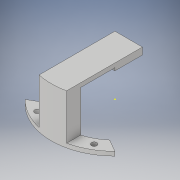
# Autodesk Inventor part: Corona_Cam_Setup_Tool._v2ipt
Saved by Autodesk Inventor 2018 (Build 220112000, 112)
## iProperties
Created: 2020-03-25
Part Number: Corona_Cam_Setup_Tool._v2ipt
Material: Generic
Document SubType Name: Modeling
Designer: Ian
Density: 1 g/cm^3
Appearance: Default
Author: Ian
Autodesk Inventor part; units mm, degrees
ref_plane "YZ Plane" through (0, 0, 0) normal (1, 0, 0) x (0, 1, 0)
ref_plane "XZ Plane" through (0, 0, 0) normal (0, 1, 0) x (-1, 0, 0)
ref_plane "XY Plane" through (0, 0, 0) normal (0, 0, 1) x (1, 0, 0)
sketch "Sketch1" plane through (0, 0, 0) normal (0, 1, 0) x (-1, 0, 0)
  circle A0 centre (-20.6375, 35.7452) radius 2
  circle A1 centre (20.6375, 35.7452) radius 2
  line L0 (0, -10) -> (-10, -10)
  line L1 (-10, -10) -> (-10, 10)
  line L2 (-10, 10) -> (10, 10)
  line L3 (10, 10) -> (10, -10)
  line L4 (10, -10) -> (0, -10)
  arc A2 (23.6974, 27.5118) -> (-23.6974, 27.5118) centre (0, 0) ccw
  arc A3 (32.696, 32.7072) -> (-32.696, 32.7072) centre (0, 0) ccw
  line L5 (20.6375, 35.7452) -> (29.2978, 40.7452) construction
  line L6 (32.696, 32.7072) -> (23.6974, 27.5118)
  arc A4 (32.696, 32.7072) -> (-32.696, 32.7072) centre (0, 0) ccw
  line L7 (0, -10) -> (0, 10)
  line L8 (-32.696, 32.7072) -> (-23.6974, 27.5118)
  arc A5 (28.2185, 30.1221) -> (-28.2185, 30.1221) centre (0, 0) ccw
  dimension "d11" = 10
  dimension "d12" = 20
  dimension "d13" = 20
  dimension "d14" = 20
  constraints: 18 end point, 9 point on circle, 6 centre point, 3 coincident, 2 perpendicular, 2 point on line, 2 symmetric about line, 1 collinear, 1 concentric, 1 midpoint
  measures "d11" distance of L0.start L0.end
  measures "d12" distance of L0.end L1.end
  measures "d13" distance of L1.end L2.end
  measures "d14" distance of L2.end L3.end
extrude "Extrusion11" add sketch "Sketch1" along normal blind 3 contours A0 A5 A1 L6 A2 L8 | A0 A5 L8 A3 L6 A1
sketch "Sketch6" plane through (0, 3, 0) normal (0, 1, 0) x (1, 0, 0)
  point P0 (0, 0)
sketch "Sketch7" plane through (0, 3, 0) normal (0, 1, 0) x (1, 0, 0)
  arc A0 (-10, -34.9065) -> (10, -34.9065) centre (0, 0) ccw
  arc A1 (-32.696, -32.7072) -> (32.696, -32.7072) centre (0, 0) ccw projected
  arc A2 (-23.6974, -27.5118) -> (23.6974, -27.5118) centre (0, 0) ccw projected
  line L0 (0, 0) -> (-10, 0)
  line L1 (10, -34.9065) -> (10, -45.1529)
  line L2 (-10, -34.9065) -> (-10, -45.1529)
  line L3 (-10, 0) -> (40, 0) construction
  arc A3 (-10, -45.1529) -> (10, -45.1529) centre (0, 0) ccw
  constraints: 8 end point, 8 point on circle, 2 centre point, 2 horizontal, 1 coincident, 1 vertical
extrude "Extrusion12" add sketch "Sketch7" along normal blind 28
sketch "Sketch8" plane through (0, 31, 0) normal (0, 1, 0) x (1, 0, 0)
  arc A0 (-10, -34.9065) -> (10, -34.9065) centre (0, 0) ccw
  arc A1 (-10, -45.1529) -> (10, -45.1529) centre (0, 0) ccw
  line L0 (10, -34.9065) -> (10, -45.1529) projected
  line L1 (10, -34.9065) -> (10, -45.1529)
  arc A2 (-23.6974, -27.5118) -> (23.6974, -27.5118) centre (0, 0) ccw projected
  line L2 (-10, -34.9065) -> (-10, -45.1529)
  arc A3 (-32.696, -32.7072) -> (32.696, -32.7072) centre (0, 0) ccw projected
  constraints: 6 point on circle, 4 end point, 2 centre point, 2 coincident, 1 collinear, 1 vertical
extrude "Extrusion13" add sketch "Sketch8" along normal blind 5
sketch "Sketch9" plane through (0, 36, 0) normal (0, 1, 0) x (1, 0, 0)
  line L0 (0, 0) -> (0, 10)
  line L1 (0, 10) -> (10, 10)
  line L2 (10, 10) -> (10, -10)
  line L3 (10, -10) -> (-10, -10)
  line L4 (-10, -10) -> (-10, 10)
  line L5 (-10, 10) -> (0, 10)
  dimension "d63" = 10
  dimension "d64" = 10
  dimension "d65" = 20
  dimension "d66" = 20
  dimension "d67" = 20
  constraints: 12 end point, 4 perpendicular, 1 point on line, 1 vertical
  measures "d63" distance of L0.start L0.end
  measures "d64" distance of L0.end L1.end
  measures "d65" distance of L1.end L2.end
  measures "d66" distance of L2.end L3.end
  measures "d67" distance of L3.end L4.end
extrude "Extrusion14" add sketch "Sketch9" against normal blind 5
sketch "Sketch10" plane through (10, 36, -10) normal (0, 0, -1) x (-1, 0, 0)
  line L0 (0, 0) -> (20, 0) projected
  line L1 (20, 0) -> (20, -3)
  line L2 (20, -33) -> (20, 0) projected
  line L3 (20, -3) -> (0, -3)
  line L4 (20, -5) -> (0, -5) projected
  line L5 (0, -33) -> (0, 0) projected
  line L6 (0, -3) -> (0, 0)
  line L7 (0, 0) -> (20, 0)
  point P0 (10, -36)
  dimension "d70" = 3
  dimension "d71" = 20
  dimension "d72" = 90
  constraints: 8 end point, 1 parallel, 1 point on line
  measures "d70" distance of L0.end L1.end
  measures "d71" distance of L1.end L3.end
  measures "d72" angle of L1 L3
extrude "Extrusion15" add sketch "Sketch10" against normal blind 50 contours L0 L1 L3 L5
body "Solid2"
